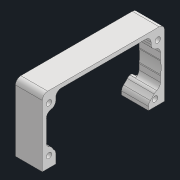
# Autodesk Inventor part: One Motor Gearbox Cover
Saved by Autodesk Inventor 2022 (Build 260153000, 153)
## iProperties
Created: 2022-09-09
Part Number: One Motor Gearbox Cover
Material: Generic
Document SubType Name: Modeling
Designer: robpl
Density: 1 g/cm^3
Appearance: Default
Author: robpl
Autodesk Inventor part; units mm, degrees
ref_plane "YZ Plane" through (0, 0, 0) normal (1, 0, 0) x (0, 1, 0)
ref_plane "XZ Plane" through (0, 0, 0) normal (0, 1, 0) x (-1, 0, 0)
ref_plane "XY Plane" through (0, 0, 0) normal (0, 0, 1) x (1, 0, 0)
sketch "Sketch2" plane through (0, 0, 0) normal (1, 0, 0) x (0, 1, 0)
  line L0 (0, 0) -> (50, 0)
  line L1 (50, 0) -> (50, 91)
  line L2 (50, 91) -> (0, 91)
  line L3 (0, 91) -> (0, 0)
  dimension "d39" = 50
  dimension "d40" = 91
  constraints: 8 end point, 2 parallel, 1 horizontal, 1 perpendicular
  measures "d39" distance of L2.end L1.end
  measures "d40" distance of L0.end L1.end
extrude "Extrusion2" add sketch "Sketch2" against normal blind 20
sketch "Sketch3" plane through (-20, 0, 0) normal (-1, 0, 0) x (0, 0, 1)
  line L0 (0, 0) -> (91, 0) projected
  line L1 (0, 50) -> (0, 0) projected
  point P0 (7, 5)
  point P1 (5, 42)
  point P2 (86, 42)
  point P3 (86, 8)
  dimension "d43" = 8
  dimension "d44" = 86
  dimension "d45" = 42
  dimension "d46" = 5
  dimension "d47" = 7
  dimension "d48" = 5
  constraints: 1 horizontal alignment, 1 vertical alignment
  measures "d43" distance from line of L0 point (86, 8)
  measures "d44" distance from line of L1 point (86, 8)
  measures "d45" distance from line of L0 point (86, 42)
  measures "d46" distance from line of L1 point (5, 42)
  measures "d47" distance from line of L1 point (7, 5)
  measures "d48" distance from line of L0 point (7, 5)
hole "Hole1" at (-20, 5, 7) at (-20, 42, 5) at (-20, 42, 86) at (-20, 8, 86) direction (1, 0, 0) diameter 4 end through all
fillet "Fillet8" radius 4 2 edges at (-10, 50, 0) (-10, 50, 91)
sketch "Sketch4" plane through (-20, 0, 0) normal (-1, 0, 0) x (0, 0, 1)
  line L0 (91, 0) -> (0, 0) projected
  line L1 (12, 0) -> (81, 0)
  line L2 (81, 13) -> (81, 0)
  line L3 (81, 13) -> (88, 13)
  line L4 (88, 13) -> (88, 37)
  line L5 (88, 37) -> (81, 37)
  line L6 (81, 37) -> (81, 47)
  line L7 (81, 47) -> (10, 47)
  line L8 (10, 47) -> (10, 37)
  line L9 (10, 37) -> (3, 37)
  line L10 (3, 37) -> (3, 10)
  line L11 (0, 46) -> (0, 0) projected
  line L12 (3, 10) -> (12, 10)
  line L13 (12, 10) -> (12, 0)
  line L14 (0, 0) -> (91, 0) projected
  dimension "d57" = 3
  dimension "d58" = 88
  dimension "d59" = 47
  dimension "d60" = 10
  dimension "d61" = 37
  dimension "d62" = 81
  dimension "d63" = 13
  dimension "d67" = 12
  dimension "d68" = 10
  constraints: 24 end point, 7 perpendicular, 6 point on line, 2 horizontal
  measures "d57" distance from line of L0.end L10
  measures "d58" distance from line of L0.end L4
  measures "d59" distance between parallel lines of L0 L7
  measures "d60" distance from line of L0.end L8
  measures "d61" distance from line of L0.end L9
  measures "d62" distance between parallel lines of L11 L6
  measures "d63" distance between parallel lines of L0 L3
  measures "d67" distance between parallel lines of L11 L13
  measures "d68" distance between parallel lines of L0 L12
extrude "Extrusion3" cut sketch "Sketch4" against normal through all
sketch "Sketch5" plane through (-20, 0, 0) normal (-1, 0, 0) x (0, 0, 1)
  circle A0 centre (25, 23) radius 22.5
  circle A1 centre (78, 14) radius 6
  point P0 (0, 0)
  dimension "d69" = 25
  dimension "d70" = 23
  dimension "d71" = 45
  dimension "d75" = 12
  dimension "d76" = 78
  dimension "d77" = 14
  constraints: 2 centre point
  measures "d69" horizontal distance of point (0, 0) A0.centre
  measures "d70" vertical distance of point (0, 0) A0.centre
  measures "d71" diameter of A0
  measures "d75" diameter of A1
  measures "d76" horizontal distance of point (0, 0) A1.centre
  measures "d77" vertical distance of point (0, 0) A1.centre
extrude "Extrusion4" cut sketch "Sketch5" against normal through all
fillet "Fillet9" radius 4 15 edges at (-10, 37, 3) (-10, 18.283, 3) (-10, 27.717, 3) (-10, 10, 3) (-10, 10, 6.6356) (-10, 4.6356, 12) (-10, 37, 7.3861) (-10, 39.7705, 10) (-10, 47, 10) (-10, 47, 81) (-10, 37, 81) (-10, 37, 88) (-10, 13, 88) (-10, 13, 83.9161) (-10, 8.8038, 81)
sketch "Sketch6" plane through (-20, 0, 0) normal (-1, 0, 0) x (0, 0, 1)
  circle A0 centre (-7.25, 21) radius 16
  point P0 (0, 0)
  dimension "d78" = 32
  dimension "d79" = 21
  dimension "d80" = 7.25
  constraints: 1 centre point
  measures "d78" diameter of A0
  measures "d79" vertical distance of point (0, 0) A0.centre
  measures "d80" horizontal distance of point (0, 0) A0.centre
extrude "Extrusion5" cut sketch "Sketch6" against normal blind 6
fillet "Fillet10" radius 2 4 edges at (-17, 35.2632, 0) (-17, 6.7368, 0) (-17, 33.2776, 3.0096) (-17, 10.3732, 4.7112)
body "Solid2"
